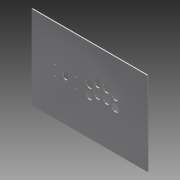
# Autodesk Inventor part: Panel_top
Saved by Autodesk Inventor 2013 (Build 170138000, 138)
## iProperties
Created: 2012-07-09
Part Number: Panel_top
Material: Aluminum 1100-H18
Document SubType Name: Modeling
Designer: mstine
Density: 1 g/cm^3
Author: mstine
Autodesk Inventor part; units mm, degrees
ref_plane "YZ Plane" through (0, 0, 0) normal (1, 0, 0) x (0, 1, 0)
ref_plane "XZ Plane" through (0, 0, 0) normal (0, 1, 0) x (-1, 0, 0)
ref_plane "XY Plane" through (0, 0, 0) normal (0, 0, 1) x (1, 0, 0)
sketch "Sketch1" plane through (0, 0, 0) normal (0, 0, 1) x (1, 0, 0)
  line L0 (-228.6, 165.1) -> (228.6, 165.1)
  line L1 (228.6, 165.1) -> (228.6, -165.1)
  line L2 (228.6, -165.1) -> (-228.6, -165.1)
  line L3 (-228.6, -165.1) -> (-228.6, 165.1)
  line L4 (-228.6, 165.1) -> (228.6, -165.1) construction
  line L5 (228.6, 165.1) -> (-228.6, -165.1) construction
  circle A0 centre (-94.9459, 0) radius 12
  circle A1 centre (0.0541, -18) radius 15
  line L6 (-94.9459, 0) -> (0.0541, 0)
  line L7 (0.0541, 0) -> (0.0541, -18)
  circle A2 centre (0.0541, 21) radius 15
  line L8 (0.0541, 21) -> (0.0541, 0)
  circle A3 centre (31.3041, 0) radius 15
  circle A4 centre (31.3041, 39) radius 15
  line L9 (0.0541, 0) -> (31.3041, 0)
  line L10 (31.3041, 0) -> (31.3041, 39)
  circle A5 centre (67.3041, 0) radius 15
  circle A6 centre (67.3041, 39) radius 15
  line L11 (31.3041, 0) -> (67.3041, 0)
  line L12 (67.3041, 0) -> (67.3041, 39)
  circle A7 centre (102.3041, -9) radius 15
  circle A8 centre (102.3041, 30) radius 15
  line L13 (67.3041, 0) -> (102.3041, 0)
  line L14 (102.3041, -9) -> (102.3041, 0)
  line L15 (102.3041, 0) -> (102.3041, 30)
  line L16 (-137.4459, 20.25) -> (-52.4459, -20.25) construction
  line L17 (-52.4459, 20.25) -> (-137.4459, -20.25) construction
  circle A9 centre (-137.4459, 20.25) radius 2.5
  circle A10 centre (-52.4459, 20.25) radius 2.5
  circle A11 centre (-52.4459, -20.25) radius 2.5
  circle A12 centre (-137.4459, -20.25) radius 2.5
  point P0 (0, 0)
  dimension "d0" = 457.2
  dimension "d2" = 330.2
  dimension "d3" = 24
  dimension "d4" = 30
  dimension "d5" = 95
  dimension "d6" = 18
  dimension "d7" = 30
  dimension "d8" = 21
  dimension "d9" = 30
  dimension "d10" = 30
  dimension "d11" = 31.25
  dimension "d12" = 39
  dimension "d13" = 30
  dimension "d14" = 30
  dimension "d15" = 36
  dimension "d16" = 39
  dimension "d17" = 30
  dimension "d18" = 30
  dimension "d20" = 35
  dimension "d21" = 9
  dimension "d22" = 30
  dimension "d27" = 85
  dimension "d28" = 40.5
  dimension "d29" = 5
  dimension "d30" = 5
  dimension "d31" = 5
  dimension "d32" = 5
  dimension "d33" = 40.5
  dimension "d34" = 85
  constraints: 36 end point, 13 centre point, 9 perpendicular, 4 midpoint, 2 collinear, 2 parallel, 1 coincident, 1 horizontal
  measures "d0" distance of L0.start L0.end
  measures "d2" distance of L2.end L0.start
  measures "d3" diameter of A0
  measures "d4" diameter of A1
  measures "d5" distance of L6.start L6.end
  measures "d6" distance of L6.end L7.end
  measures "d7" diameter of A2
  measures "d8" distance of L8.start L6.end
  measures "d9" diameter of A3
  measures "d10" diameter of A4
  measures "d11" distance of L6.end L9.end
  measures "d12" distance of L9.end L10.end
  measures "d13" diameter of A5
  measures "d14" diameter of A6
  measures "d15" distance of L9.end L11.end
  measures "d16" distance of L11.end L12.end
  measures "d17" diameter of A7
  measures "d18" diameter of A8
  measures "d20" distance of L11.end L13.end
  measures "d21" distance of L14.start L13.end
  measures "d22" distance of L13.end L15.end
  measures "d27" distance of L16.end L17.end
  measures "d28" distance of L17.start L16.end
  measures "d29" diameter of A9
  measures "d30" diameter of A10
  measures "d31" diameter of A11
  measures "d32" diameter of A12
  measures "d33" distance of A12.centre L16.start
  measures "d34" distance of L17.start L16.start
extrude "Extrusion2" add sketch "Sketch1" along normal blind 4
body "Solid2"
